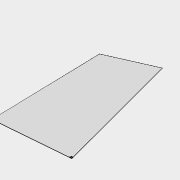
# Autodesk Inventor part: Drilled plate
Saved by Autodesk Inventor 2020.1 (Build 241239000, 239)
## iProperties
Created: 2019-09-15
Part Number: Drilled plate
Material: Generic
Document SubType Name: Modeling
Designer: thomastremblay
Density: 1 g/cm^3
Appearance: Default
Author: thomastremblay
Autodesk Inventor part; units mm, degrees
ref_plane "YZ Plane" through (0, 0, 0) normal (1, 0, 0) x (0, 1, 0)
ref_plane "XZ Plane" through (0, 0, 0) normal (0, 1, 0) x (-1, 0, 0)
ref_plane "XY Plane" through (0, 0, 0) normal (0, 0, 1) x (1, 0, 0)
sketch "Sketch1" plane through (0, 0, 0) normal (0, 0, 1) x (1, 0, 0)
  line L0 (0, 0) -> (2438.4, 0)
  line L1 (2438.4, 0) -> (2438.4, 1219.2)
  line L2 (2438.4, 1219.2) -> (0, 1219.2)
  line L3 (0, 1219.2) -> (0, 0)
  dimension "d0" = 2438.4
  dimension "d1" = 1219.2
  constraints: 8 end point, 2 parallel, 1 horizontal, 1 perpendicular
  measures "d0" distance of L2.end L1.end
  measures "d1" distance of L1.end L0.end
extrude "Extrusion1" add sketch "Sketch1" along normal blind 6
sketch "Sketch2" plane through (0, 0, 6) normal (0, 0, 1) x (1, 0, 0)
  line L0 (16.8875, 6.5) -> (16.8875, 19.5) construction
  line L1 (16.8875, 19.5) -> (5.6292, 13) construction
  line L2 (5.6292, 13) -> (16.8875, 6.5) construction
  line L3 (0, 0) -> (2438.4, 0) projected
  line L4 (0, 1219.2) -> (0, 0) projected
  line L5 (5.6292, 13) -> (5.6292, 26) construction
  line L6 (5.6292, 26) -> (16.8875, 19.5) construction
  dimension "Y_space" = 13
  dimension "d5" = 6.5
  dimension "d6" = 5.6292
  dimension "X_space" = 11.2583
  constraints: 10 end point, 3 equal length, 2 vertical
  measures "Y_space" distance of L0.start L0.end
  measures "d5" distance from line of L3 L0.start
  measures "d6" distance from line of L4 L1.end
  measures "X_space" horizontal distance of L1.end L0.start
hole "Hole1" at (5.6292, 13, 6) at (16.8875, 19.5, 6) at (16.8875, 6.5, 6) at (5.6292, 26, 6) direction (0, 0, -1) diameter 10 end through all
equation "\"d5\" = 0.5 * Y_space"
equation "\"d6\" = 0.5 * X_space"
body "Solid1"
